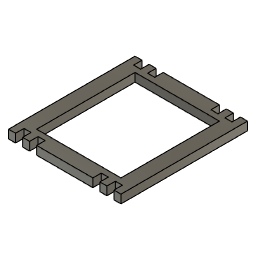
Carrier Top Piece v3 (Autodesk Fusion 360 design; units mm, degrees)
Autodesk Fusion 360 part; units mm, degrees
sketch "Sketch1" plane through (0, 0, 0) normal (0, 0, 1) x (1, 0, 0)
  line L0 (40, 45) -> (-40, 45)
  line L1 (-40, 45) -> (-40, -45)
  line L2 (-40, -45) -> (40, -45)
  line L3 (40, -45) -> (40, 45)
  line L4 (40, 45) -> (-40, -45) construction
  line L5 (-40, 45) -> (40, -45) construction
  line L6 (30, 35) -> (-30, 35)
  line L7 (-30, 35) -> (-30, -35)
  line L8 (-30, -35) -> (30, -35)
  line L9 (30, -35) -> (30, 35)
  line L10 (30, 35) -> (-30, -35) construction
  line L11 (-30, 35) -> (30, -35) construction
  dimension "d1" = 80
  dimension "d2" = 90
  dimension "d3" = 60
  dimension "d6" = 10
  constraint horizontal L0
  constraint perpendicular L0 L1
  constraint parallel L0 L2
  constraint parallel L1 L3
  constraint coincident L4 origin
  constraint coincident L5 origin
  constraint horizontal L6
  constraint perpendicular L6 L7
  constraint parallel L6 L8
  constraint parallel L7 L9
  constraint coincident L10 origin
  constraint coincident L11 origin
  measures "d1" distance of L1.end L2.end
  measures "d2" distance of L0.end L1.end
  measures "d3" distance of L7.end L8.end
  measures "d6" distance of L0 L6
extrude "Extrude1" add sketch "Sketch1" along normal blind 6
sketch "Sketch2" plane through (0, 0, 6) normal (0, 0, 1) x (-1, 0, 0)
  line L0 (-30, -35) -> (-30, 35)
  line L1 (-30, 35) -> (30, 35)
  line L2 (30, 35) -> (30, -35)
  line L3 (30, -35) -> (-30, -35)
  line L4 (-40, 45) -> (-40, -45)
  line L5 (-40, -45) -> (40, -45)
  line L6 (40, -45) -> (40, 45)
  line L7 (40, 45) -> (-40, 45)
  line L8 (-40, 45) -> (-35, 45) construction
  line L9 (-35, 45) -> (-35, 39) construction
  line L10 (-35, 39) -> (-40, 39) construction
  line L11 (-40, 39) -> (-40, 45) construction
  line L12 (-35, 45) -> (-30, 45) construction
  line L13 (-30, 45) -> (-30, 39) construction
  line L14 (-30, 39) -> (-35, 39) construction
  line L15 (-35, 39) -> (-35, 45) construction
  line L16 (-30, 45) -> (-25, 45) construction
  line L17 (-25, 45) -> (-25, 39) construction
  line L18 (-25, 39) -> (-30, 39) construction
  line L19 (-30, 39) -> (-30, 45) construction
  line L20 (-25, 45) -> (-20, 45) construction
  line L21 (-20, 45) -> (-20, 39) construction
  line L22 (-20, 39) -> (-25, 39) construction
  line L23 (-25, 39) -> (-25, 45) construction
  line L24 (-30, 39) -> (-35, 39)
  line L25 (-35, 39) -> (-35, 45)
  line L26 (-35, 45) -> (-30, 45)
  line L27 (-30, 45) -> (-30, 39)
  line L28 (-20, 39) -> (-25, 39)
  line L29 (-25, 39) -> (-25, 45)
  line L30 (-25, 45) -> (-20, 45)
  line L31 (-20, 45) -> (-20, 39)
  line L32 (40, 45) -> (35, 45) construction
  line L33 (35, 45) -> (35, 39) construction
  line L34 (35, 39) -> (40, 39) construction
  line L35 (40, 39) -> (40, 45) construction
  line L36 (35, 39) -> (30, 39)
  line L37 (30, 39) -> (30, 45)
  line L38 (30, 45) -> (35, 45)
  line L39 (35, 45) -> (35, 39)
  line L40 (30, 39) -> (25, 39) construction
  line L41 (25, 39) -> (25, 45) construction
  line L42 (25, 45) -> (30, 45) construction
  line L43 (30, 45) -> (30, 39) construction
  line L44 (25, 39) -> (20, 39)
  line L45 (20, 39) -> (20, 45)
  line L46 (20, 45) -> (25, 45)
  line L47 (25, 45) -> (25, 39)
  constraint horizontal L8
  constraint vertical L9
  constraint horizontal L10
  constraint vertical L11
  constraint coincident L4.start L7.end
  constraint horizontal L12
  constraint vertical L13
  constraint horizontal L14
  constraint vertical L15
  constraint horizontal L16
  constraint vertical L17
  constraint horizontal L18
  constraint vertical L19
  constraint horizontal L20
  constraint vertical L21
  constraint horizontal L22
  constraint vertical L23
  constraint horizontal L24
  constraint vertical L25
  constraint horizontal L26
  constraint vertical L27
  constraint horizontal L28
  constraint vertical L29
  constraint horizontal L30
  constraint vertical L31
  constraint horizontal L32
  constraint vertical L33
  constraint horizontal L34
  constraint vertical L35
  constraint coincident L6.end L7.start
  constraint horizontal L36
  constraint vertical L37
  constraint horizontal L38
  constraint vertical L39
  constraint coincident L7 L37.end
  constraint horizontal L40
  constraint vertical L41
  constraint horizontal L42
  constraint vertical L43
  constraint coincident L7 L41.end
  constraint horizontal L44
  constraint vertical L45
  constraint horizontal L46
  constraint vertical L47
  constraint coincident L7 L45.end
extrude "Extrude2" cut sketch "Sketch2" against normal blind 6 contours L7 L24 L25 L26 L27 | L7 L28 L29 L30 L31
ref_plane "WorkPlane1" through (0, 0, 0) normal (0, 1, 0) x (0, 0, 1)
ref_plane "WorkPlane2" through (0, 0, 0) normal (1, 0, 0) x (0, 1, 0)
extrude "Extrude3" cut sketch "Sketch2" against normal blind 6 contours L7 L24 L25 L26 L27 | L7 L28 L29 L30 L31 | L7 L36 L37 L38 L39 | L7 L44 L45 L46 L47
mirror "Mirror3" about plane through (0, 0, 0) normal (0, 1, 0) of "Extrude3"
